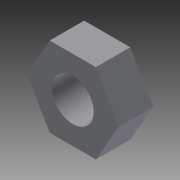
# Autodesk Inventor part: SensorNut-M3
Saved by Autodesk Inventor 2015 (Build 190159000, 159)
## iProperties
Created: 2017-03-05
Part Number: SensorNut-M3
Material: Generic
Document SubType Name: Modeling
Designer: 1esh9
Density: 1 g/cm^3
Appearance: Default
Author: 1esh9
Autodesk Inventor part; units mm, degrees
ref_plane "YZ Plane" through (0, 0, 0) normal (1, 0, 0) x (0, 1, 0)
ref_plane "XZ Plane" through (0, 0, 0) normal (0, 1, 0) x (-1, 0, 0)
ref_plane "XY Plane" through (0, 0, 0) normal (0, 0, 1) x (1, 0, 0)
sketch "Sketch1" plane through (0, 0, 0) normal (0, 1, 0) x (-1, 0, 0)
  line L0 (3.1466, 0) -> (1.5733, -2.725)
  line L1 (1.5733, -2.725) -> (-1.5733, -2.725)
  line L2 (-1.5733, -2.725) -> (-3.1466, 0)
  line L3 (-3.1466, 0) -> (-1.5733, 2.725)
  line L4 (-1.5733, 2.725) -> (1.5733, 2.725)
  line L5 (1.5733, 2.725) -> (3.1466, 0)
  circle A0 centre (0, 0) radius 1.425
  dimension "d0" = 5.45
  dimension "d3" = 2.85
  constraints: 12 end point, 2 coincident, 1 centre point, 13 other
  measures "d0" distance between parallel lines of L3 L0
  measures "d3" diameter of A0
extrude "Extrusion1" add sketch "Sketch1" along normal blind 2.35
body "Solid1"
